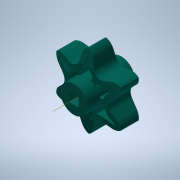
# Autodesk Inventor part: 276-2252.html
Saved by Autodesk Inventor 2020 (Build 240168000, 168)
## iProperties
Created: 2012-02-28
Part Number: 276-2252.html
Document SubType Name: Modeling
Designer: Autodesk Inc.
Density: 1.42 g/cm^3
Material: Acetal Resin, White
Catalog Web Link: http://www.vexrobotics.com/276-2252.html#
Vendor: VEX
Mass: 3.55844 g
Surface Area: 16.0324 cm^2
Volume: 2.50594 cm^3
Appearance: VEX Gears Green
Category: Motion
Company: Autodesk Inc.
Author: Autodesk Inc.
Autodesk Inventor part; units mm, degrees
ref_plane "YZ Plane" through (0, 0, 0) normal (1, 0, 0) x (0, 1, 0)
ref_plane "XZ Plane" through (0, 0, 0) normal (0, 1, 0) x (-1, 0, 0)
ref_plane "XY Plane" through (0, 0, 0) normal (0, 0, 1) x (1, 0, 0)
sketch "Sketch1" plane through (0, 0, 0) normal (0, 0, 1) x (1, 0, 0)
  arc A0 (-7.9913, 6.691) -> (-10.7412, 6.2014) centre (-8.8664, 3.639) ccw
  line L0 (-7.9913, 6.691) -> (-5.6103, 6.0082)
  arc A1 (-5.6103, 6.0082) -> (-2.3981, 7.8628) centre (-4.8997, 8.4865) ccw
  line L1 (-2.3981, 7.8628) -> (-1.7989, 10.2662)
  arc A2 (0, 12.4028) -> (-1.7989, 10.2662) centre (1.2818, 9.4981) ccw
  arc A3 (1.7989, 10.2662) -> (0, 12.4028) centre (-1.2818, 9.4981) ccw
  line L2 (1.7989, 10.2662) -> (2.3981, 7.8628)
  arc A4 (2.3981, 7.8628) -> (5.6103, 6.0082) centre (4.8997, 8.4865) ccw
  line L3 (5.6103, 6.0082) -> (7.9913, 6.691)
  arc A5 (10.7412, 6.2014) -> (7.9913, 6.691) centre (8.8664, 3.639) ccw
  arc A6 (9.7902, 3.5752) -> (10.7412, 6.2014) centre (7.5847, 5.8591) ccw
  line L4 (9.7902, 3.5752) -> (8.0084, 1.8545)
  arc A7 (8.0084, 1.8545) -> (8.0084, -1.8545) centre (9.7993, 0) ccw
  line L5 (8.0084, -1.8545) -> (9.7902, -3.5752)
  arc A8 (10.7412, -6.2014) -> (9.7902, -3.5752) centre (7.5847, -5.8591) ccw
  arc A9 (7.9913, -6.691) -> (10.7412, -6.2014) centre (8.8664, -3.639) ccw
  line L6 (7.9913, -6.691) -> (5.6103, -6.0082)
  arc A10 (5.6103, -6.0082) -> (2.3981, -7.8628) centre (4.8997, -8.4865) ccw
  line L7 (2.3981, -7.8628) -> (1.7989, -10.2662)
  arc A11 (0, -12.4028) -> (1.7989, -10.2662) centre (-1.2818, -9.4981) ccw
  arc A12 (-1.7989, -10.2662) -> (0, -12.4028) centre (1.2818, -9.4981) ccw
  line L8 (-1.7989, -10.2662) -> (-2.3981, -7.8628)
  arc A13 (-2.3981, -7.8628) -> (-5.6103, -6.0082) centre (-4.8997, -8.4865) ccw
  line L9 (-5.6103, -6.0082) -> (-7.9913, -6.691)
  arc A14 (-10.7412, -6.2014) -> (-7.9913, -6.691) centre (-8.8664, -3.639) ccw
  arc A15 (-9.7902, -3.5752) -> (-10.7412, -6.2014) centre (-7.5847, -5.8591) ccw
  line L10 (-9.7902, -3.5752) -> (-8.0084, -1.8545)
  arc A16 (-8.0084, -1.8545) -> (-8.0084, 1.8545) centre (-9.7993, 0) ccw
  line L11 (-8.0084, 1.8545) -> (-9.7902, 3.5752)
  arc A17 (-10.7412, 6.2014) -> (-9.7902, 3.5752) centre (-7.5847, 5.8591) ccw
  line L12 (-1.5875, 1.5875) -> (-1.5875, -1.5875)
  line L13 (-1.5875, -1.5875) -> (1.5875, -1.5875)
  line L14 (1.5875, -1.5875) -> (1.5875, 1.5875)
  line L15 (1.5875, 1.5875) -> (-1.5875, 1.5875)
  point P0 (0, 0)
  point P1 (0, 0)
  constraints: 36 point on circle, 32 end point, 18 centre point
extrude "Extrusion1" add sketch "Sketch1" along normal mid plane 7.62 contours L0 A1 L1 A2 A3 L2 A4 L3 A5 A6 L4 A7 L5 A8 A9 L6 A10 L7 A11 A12 L8 A13 L9 A14 A15 L10 A16 L11 A17 A0 | L15 L14 L13 L12
sketch "Sketch2" plane through (0, 0, 3.81) normal (0, 0, 1) x (1, 0, 0)
  circle A0 centre (0, 0) radius 4.4958
  dimension "d2" = 8.9916
  constraints: 1 centre point, 1 coincident
  measures "d2" diameter of A0
extrude "Extrusion2" add sketch "Sketch2" along normal blind 4.1402
mirror "Mirror1" about plane through (0, 0, 0) normal (0, 0, 1) of "Extrusion2"
extrude "Extrusion3" cut sketch "Sketch1" against normal up to surface (15.9004 mm away) from surface at 7.9502 contours L15 L14 L13 L12
sketch "Sketch3" plane through (0, 0, 3.81) normal (0, 0, 1) x (1, 0, 0)
  line L0 (-7.9913, 6.691) -> (-5.6103, 6.0082) projected
  arc A0 (-7.9913, 6.691) -> (-10.7412, 6.2014) centre (-8.8664, 3.639) ccw projected
  arc A1 (-10.7412, 6.2014) -> (-9.7902, 3.5752) centre (-7.5847, 5.8591) ccw projected
  line L1 (-8.0084, 1.8545) -> (-9.7902, 3.5752) projected
  arc A2 (-8.0084, -1.8545) -> (-8.0084, 1.8545) centre (-9.7993, 0) ccw projected
  line L2 (-9.7902, -3.5752) -> (-8.0084, -1.8545) projected
  arc A3 (-9.7902, -3.5752) -> (-10.7412, -6.2014) centre (-7.5847, -5.8591) ccw projected
  arc A4 (-10.7412, -6.2014) -> (-7.9913, -6.691) centre (-8.8664, -3.639) ccw projected
  line L3 (-5.6103, -6.0082) -> (-7.9913, -6.691) projected
  arc A5 (-2.3981, -7.8628) -> (-5.6103, -6.0082) centre (-4.8997, -8.4865) ccw projected
  line L4 (-1.7989, -10.2662) -> (-2.3981, -7.8628) projected
  arc A6 (-1.7989, -10.2662) -> (0, -12.4028) centre (1.2818, -9.4981) ccw projected
  arc A7 (0, -12.4028) -> (1.7989, -10.2662) centre (-1.2818, -9.4981) ccw projected
  line L5 (2.3981, -7.8628) -> (1.7989, -10.2662) projected
  arc A8 (5.6103, -6.0082) -> (2.3981, -7.8628) centre (4.8997, -8.4865) ccw projected
  line L6 (7.9913, -6.691) -> (5.6103, -6.0082) projected
  arc A9 (7.9913, -6.691) -> (10.7412, -6.2014) centre (8.8664, -3.639) ccw projected
  arc A10 (10.7412, -6.2014) -> (9.7902, -3.5752) centre (7.5847, -5.8591) ccw projected
  line L7 (8.0084, -1.8545) -> (9.7902, -3.5752) projected
  arc A11 (8.0084, 1.8545) -> (8.0084, -1.8545) centre (9.7993, 0) ccw projected
  line L8 (9.7902, 3.5752) -> (8.0084, 1.8545) projected
  arc A12 (9.7902, 3.5752) -> (10.7412, 6.2014) centre (7.5847, 5.8591) ccw projected
  arc A13 (10.7412, 6.2014) -> (7.9913, 6.691) centre (8.8664, 3.639) ccw projected
  line L9 (5.6103, 6.0082) -> (7.9913, 6.691) projected
  arc A14 (2.3981, 7.8628) -> (5.6103, 6.0082) centre (4.8997, 8.4865) ccw projected
  line L10 (1.7989, 10.2662) -> (2.3981, 7.8628) projected
  arc A15 (1.7989, 10.2662) -> (0, 12.4028) centre (-1.2818, 9.4981) ccw projected
  arc A16 (0, 12.4028) -> (-1.7989, 10.2662) centre (1.2818, 9.4981) ccw projected
  line L11 (-2.3981, 7.8628) -> (-1.7989, 10.2662) projected
  arc A17 (-5.6103, 6.0082) -> (-2.3981, 7.8628) centre (-4.8997, 8.4865) ccw projected
  circle A18 centre (0, 0) radius 5.0673 projected
  circle A19 centre (0, 0) radius 7.6454
  dimension "d8" = 15.2908
  constraints: 1 centre point, 1 coincident
  measures "d8" diameter of A19
sketch "Sketch4" plane through (0, 0, 0) normal (1, 0, 0) x (0, 1, 0)
  line L0 (7.6454, 3.81) -> (-7.6454, 3.81) projected
  line L1 (12.4028, 3.81) -> (12.4028, 2.9972)
  line L2 (12.4028, 2.9972) -> (7.6454, 3.81)
  line L3 (7.6454, 3.81) -> (12.4028, 3.81)
  line L4 (0, -0.762) -> (0, 4.572) projected
  point P0 (0, 0)
  dimension "d9" = 0.8128
  constraints: 6 end point
  measures "d9" distance of L1.start L1.end
revolve "Revolution1" cut sketch "Sketch4" angle 360 about axis through (0, 0, -10) along (0, 0, 1)
mirror "Mirror2" about plane through (0, 0, 0) normal (0, 0, 1) of "Revolution1"
sketch "Sketch5" plane through (0, 0, 3.81) normal (0, 0, 1) x (1, 0, 0)
  circle A0 centre (0, 0) radius 4.2
  line L0 (1.5875, 1.5875) -> (-1.5875, 1.5875)
  line L1 (1.5875, -1.5875) -> (1.5875, 1.5875)
  line L2 (-1.5875, -1.5875) -> (1.5875, -1.5875)
  line L3 (-1.5875, 1.5875) -> (-1.5875, -1.5875)
  line L4 (1.5875, -1.5875) -> (1.5875, 1.5875)
  line L5 (1.5875, 1.5875) -> (-1.5875, 1.5875)
  line L6 (-1.5875, 1.5875) -> (-1.5875, -1.5875)
  line L7 (-1.5875, -1.5875) -> (1.5875, -1.5875)
  circle A1 centre (0, 0) radius 4.2
  line L8 (9.0737, 4.9685) -> (7.2002, 3.1592)
  arc A2 (7.715, 1.5173) -> (7.2002, 3.1592) centre (0, 0) ccw
  spline S0 degree 3 poles (8.0084, 1.8545) (7.9726, 1.8199) (7.9378, 1.7843) (7.904, 1.7477) (7.8703, 1.7111) (7.8377, 1.6736) (7.8061, 1.6352) (7.7746, 1.5967) (7.7442, 1.5574) (7.715, 1.5173) knots 0 0 0 0 0.333333 0.333333 0.333333 0.666667 0.666667 0.666667 1 1 1 1
  line L9 (9.7902, 3.5752) -> (8.0084, 1.8545)
  spline S1 degree 3 poles (10.7537, 6.0542) (10.7649, 5.8724) (10.7604, 5.6896) (10.7402, 5.5082) (10.7201, 5.3269) (10.6842, 5.1472) (10.6331, 4.9717) (10.582, 4.7962) (10.5157, 4.6249) (10.435, 4.4605) (10.3544, 4.2961) (10.2594, 4.1386) (10.1514, 3.9902) (10.0434, 3.8419) (9.9224, 3.7029) (9.7902, 3.5752) knots 0 0 0 0 0.2 0.2 0.2 0.4 0.4 0.4 0.6 0.6 0.6 0.8 0.8 0.8 1 1 1 1
  ellipse E0 centre (10.4543, 6.0358) end of major axis (10.6042, 5.776) minor radius 0.2999 (10.7537, 6.0542) -> (10.6199, 6.2859) ccw
  spline S2 degree 3 poles (10.6199, 6.2859) (10.2987, 6.4986) (9.9401, 6.6495) (9.1019, 6.8432) (8.5734, 6.8415) (8.049, 6.7071) (8.0201, 6.6992) (7.9913, 6.691) knots 0 0 0 0 0.414162 0.414162 0.967573 0.967573 1 1 1 1
  spline S3 degree 3 poles (7.9913, 6.691) (7.7038, 6.6085) (7.144, 6.448) (6.3504, 6.2205) (5.8519, 6.0775) (5.6103, 6.0082) knots 0 0 0 0 0.333333 0.666667 1 1 1 1
  spline S4 degree 3 poles (5.1715, 5.9227) (5.2209, 5.928) (5.2701, 5.9346) (5.3192, 5.9427) (5.3682, 5.9508) (5.4171, 5.9603) (5.4656, 5.9712) (5.5141, 5.9822) (5.5624, 5.9945) (5.6103, 6.0082) knots 0 0 0 0 0.333333 0.333333 0.333333 0.666667 0.666667 0.666667 1 1 1 1
  arc A3 (6.3361, 4.6559) -> (5.1715, 5.9227) centre (0, 0) ccw
  spline S5 degree 3 poles (6.3361, 4.6559) (6.5468, 4.7163) (6.9811, 4.8409) (7.6702, 5.0385) (8.1556, 5.1776) (8.4048, 5.2491) knots 0 0 0 0 0.333333 0.666667 1 1 1 1
  spline S6 degree 3 poles (8.9441, 5.3122) (8.8534, 5.3164) (8.7624, 5.3132) (8.6721, 5.3027) (8.5819, 5.2921) (8.4923, 5.2742) (8.4048, 5.2491) knots 0 0 0 0 0.5 0.5 0.5 1 1 1 1
  spline S7 degree 3 poles (8.9441, 5.3122) (8.9583, 5.3115) (8.9723, 5.3093) (9.0099, 5.2995) (9.0348, 5.2877) (9.0777, 5.2549) (9.0957, 5.2339) (9.1211, 5.1896) (9.13, 5.1634) (9.1366, 5.1098) (9.1341, 5.0824) (9.1203, 5.0334) (9.1079, 5.0087) (9.0857, 4.9809) (9.0799, 4.9745) (9.0737, 4.9685) knots 0 0 0 0 0.091575 0.091575 0.26196 0.26196 0.432344 0.432344 0.602729 0.602729 0.773114 0.773114 0.945021 0.945021 1 1 1 1
  line L10 (5.549, -0.75) -> (4.6837, -0.75)
  arc A4 (5.8402, -0.9781) -> (5.549, -0.75) centre (5.549, -1.05) ccw
  arc A5 (5.8402, -0.9781) -> (6.9664, -2.9335) centre (9.7993, 0) ccw
  line L11 (7.2002, -3.1592) -> (6.9664, -2.9335)
  arc A6 (7.2002, -3.1592) -> (7.715, -1.5173) centre (0, 0) ccw
  arc A7 (7.715, 1.5173) -> (7.715, -1.5173) centre (9.7993, 0) ccw
  arc A8 (7.715, 1.5173) -> (7.2002, 3.1592) centre (0, 0) ccw
  line L12 (7.2002, 3.1592) -> (6.9664, 2.9335)
  arc A9 (6.9664, 2.9335) -> (5.8402, 0.9781) centre (9.7993, 0) ccw
  arc A10 (5.549, 0.75) -> (5.8402, 0.9781) centre (5.549, 1.05) ccw
  line L13 (4.6837, 0.75) -> (5.549, 0.75)
  arc A11 (4.391, 0.9844) -> (4.6837, 0.75) centre (4.6837, 1.05) ccw
  arc A12 (4.391, -0.9844) -> (4.391, 0.9844) centre (0, 0) ccw
  arc A13 (4.6837, -0.75) -> (4.391, -0.9844) centre (4.6837, -1.05) ccw
  spline S8 degree 3 poles (8.4048, -5.2491) (8.4923, -5.2742) (8.5818, -5.2921) (8.672, -5.3027) (8.7623, -5.3132) (8.8534, -5.3164) (8.9441, -5.3122) knots 0 0 0 0 0.5 0.5 0.5 1 1 1 1
  line L14 (8.4048, -5.2491) -> (6.3361, -4.6559)
  arc A14 (5.1715, -5.9227) -> (6.3361, -4.6559) centre (0, 0) ccw
  spline S9 degree 3 poles (5.6103, -6.0082) (5.5624, -5.9945) (5.5141, -5.9822) (5.4656, -5.9712) (5.4171, -5.9603) (5.3682, -5.9508) (5.3192, -5.9427) (5.2701, -5.9346) (5.2209, -5.928) (5.1715, -5.9227) knots 0 0 0 0 0.333333 0.333333 0.333333 0.666667 0.666667 0.666667 1 1 1 1
  line L15 (7.9913, -6.691) -> (5.6103, -6.0082)
  spline S10 degree 3 poles (10.6199, -6.2859) (10.2987, -6.4986) (9.9401, -6.6495) (9.1019, -6.8432) (8.5734, -6.8415) (8.049, -6.7071) (8.0201, -6.6992) (7.9913, -6.691) knots 0 0 0 0 0.414162 0.414162 0.967573 0.967573 1 1 1 1
  ellipse E1 centre (10.4543, -6.0358) end of major axis (10.3043, -6.2955) minor radius 0.2999 (10.6199, -6.2859) -> (10.7537, -6.0542) ccw
  spline S11 degree 3 poles (9.7902, -3.5752) (9.9224, -3.7029) (10.0434, -3.8419) (10.1514, -3.9903) (10.2594, -4.1386) (10.3544, -4.2961) (10.4351, -4.4605) (10.5157, -4.6249) (10.582, -4.7962) (10.6331, -4.9717) (10.6842, -5.1472) (10.7201, -5.3269) (10.7402, -5.5083) (10.7604, -5.6896) (10.7649, -5.8724) (10.7537, -6.0542) knots 0 0 0 0 0.2 0.2 0.2 0.4 0.4 0.4 0.6 0.6 0.6 0.8 0.8 0.8 1 1 1 1
  line L16 (9.7902, -3.5752) -> (8.0084, -1.8545)
  spline S12 degree 3 poles (7.715, -1.5173) (7.7442, -1.5574) (7.7746, -1.5967) (7.8061, -1.6352) (7.8377, -1.6736) (7.8703, -1.7111) (7.904, -1.7477) (7.9378, -1.7843) (7.9726, -1.8199) (8.0084, -1.8545) knots 0 0 0 0 0.333333 0.333333 0.333333 0.666667 0.666667 0.666667 1 1 1 1
  arc A15 (7.2002, -3.1592) -> (7.715, -1.5173) centre (0, 0) ccw
  spline S13 degree 3 poles (7.2002, -3.1592) (7.3872, -3.3398) (7.7753, -3.7147) (8.3989, -4.3169) (8.844, -4.7467) (9.0737, -4.9685) knots 0 0 0 0 0.333333 0.666667 1 1 1 1
  spline S14 degree 3 poles (9.0737, -4.9685) (9.0799, -4.9745) (9.0857, -4.9809) (9.1079, -5.0087) (9.1203, -5.0334) (9.1341, -5.0824) (9.1366, -5.1098) (9.13, -5.1634) (9.1211, -5.1896) (9.0957, -5.2339) (9.0777, -5.2549) (9.0348, -5.2877) (9.0099, -5.2995) (8.9723, -5.3093) (8.9583, -5.3115) (8.9441, -5.3122) knots 0 0 0 0 0.054979 0.054979 0.226886 0.226886 0.397271 0.397271 0.567656 0.567656 0.73804 0.73804 0.908425 0.908425 1 1 1 1
  arc A16 (1.343, -4.2949) -> (3.048, -3.3105) centre (0, 0) ccw
  arc A17 (1.6924, -4.4312) -> (1.343, -4.2949) centre (1.4325, -4.5812) ccw
  line L17 (2.125, -5.1806) -> (1.6924, -4.4312)
  arc A18 (2.0731, -5.5468) -> (2.125, -5.1806) centre (1.8652, -5.3306) ccw
  arc A19 (2.0731, -5.5468) -> (0.9427, -7.4999) centre (4.8997, -8.4865) ccw
  line L18 (0.8641, -7.8151) -> (0.9427, -7.4999)
  arc A20 (0.8641, -7.8151) -> (2.5435, -7.44) centre (0, 0) ccw
  arc A21 (5.1715, -5.9227) -> (2.5435, -7.44) centre (4.8997, -8.4865) ccw
  arc A22 (5.1715, -5.9227) -> (6.3361, -4.6559) centre (0, 0) ccw
  line L19 (6.3361, -4.6559) -> (6.0237, -4.5663)
  arc A23 (6.0237, -4.5663) -> (3.7671, -4.5688) centre (4.8997, -8.4865) ccw
  arc A24 (3.424, -4.4306) -> (3.7671, -4.5688) centre (3.6838, -4.2806) ccw
  line L20 (2.9914, -3.6812) -> (3.424, -4.4306)
  arc A25 (3.048, -3.3105) -> (2.9914, -3.6812) centre (3.2512, -3.5312) ccw
  spline S15 degree 3 poles (-0.3435, -9.9033) (-0.3233, -9.9842) (-0.2969, -10.064) (-0.2383, -10.2051) (-0.2078, -10.2671) (-0.1738, -10.3269) knots 0 0 0 0 0.548983 0.548983 1 1 1 1
  line L21 (-0.3435, -9.9033) -> (-0.8641, -7.8151)
  arc A26 (-2.5435, -7.44) -> (-0.8641, -7.8151) centre (0, 0) ccw
  spline S16 degree 3 poles (-2.3981, -7.8628) (-2.4102, -7.8144) (-2.4236, -7.7665) (-2.4384, -7.719) (-2.4533, -7.6715) (-2.4694, -7.6244) (-2.487, -7.5779) (-2.5045, -7.5314) (-2.5233, -7.4854) (-2.5435, -7.44) knots 0 0 0 0 0.333333 0.333333 0.333333 0.666667 0.666667 0.666667 1 1 1 1
  line L22 (-1.7989, -10.2662) -> (-2.3981, -7.8628)
  spline S17 degree 3 poles (-0.1338, -12.34) (-0.4786, -12.1683) (-0.7886, -11.9332) (-1.3754, -11.3041) (-1.6382, -10.8456) (-1.784, -10.3242) (-1.7917, -10.2952) (-1.7989, -10.2662) knots 0 0 0 0 0.414162 0.414162 0.967573 0.967573 1 1 1 1
  ellipse E2 centre (0, -12.0716) end of major axis (-0.2999, -12.0715) minor radius 0.2999 (-0.1338, -12.34) -> (0.1338, -12.34) ccw
  spline S18 degree 3 poles (0.1338, -12.34) (0.4786, -12.1683) (0.7886, -11.9332) (1.3754, -11.3041) (1.6382, -10.8456) (1.784, -10.3242) (1.7917, -10.2952) (1.7989, -10.2662) knots 0 0 0 0 0.414162 0.414162 0.967573 0.967573 1 1 1 1
  spline S19 degree 3 poles (1.7989, -10.2662) (1.8713, -9.9759) (2.0121, -9.4109) (2.2119, -8.6098) (2.3373, -8.1066) (2.3981, -7.8628) knots 0 0 0 0 0.333333 0.666667 1 1 1 1
  spline S20 degree 3 poles (2.5435, -7.44) (2.5233, -7.4854) (2.5045, -7.5314) (2.487, -7.5779) (2.4694, -7.6244) (2.4533, -7.6715) (2.4384, -7.719) (2.4236, -7.7665) (2.4102, -7.8144) (2.3981, -7.8628) knots 0 0 0 0 0.333333 0.333333 0.333333 0.666667 0.666667 0.666667 1 1 1 1
  arc A27 (0.8641, -7.8151) -> (2.5435, -7.44) centre (0, 0) ccw
  line L23 (0.8641, -7.8151) -> (0.3435, -9.9033)
  spline S21 degree 3 poles (0.1738, -10.3269) (0.2078, -10.2671) (0.2383, -10.2051) (0.2969, -10.064) (0.3233, -9.9842) (0.3435, -9.9033) knots 0 0 0 0 0.451017 0.451017 1 1 1 1
  spline S22 degree 3 poles (0.1738, -10.3269) (0.1621, -10.3473) (0.1468, -10.3657) (0.1289, -10.3808) (0.1109, -10.396) (0.0903, -10.4079) (0.0683, -10.4159) (0.0463, -10.4239) (0.023, -10.4279) (-0.0003, -10.4279) (-0.0236, -10.4279) (-0.0469, -10.4237) (-0.0688, -10.4157) (-0.0907, -10.4077) (-0.1112, -10.3958) (-0.129, -10.3807) (-0.1469, -10.3656) (-0.1622, -10.3473) (-0.1738, -10.3269) knots 0 0 0 0 0.166667 0.166667 0.166667 0.333333 0.333333 0.333333 0.5 0.5 0.5 0.666667 0.666667 0.666667 0.833333 0.833333 0.833333 1 1 1 1
  arc A28 (-3.048, -3.3105) -> (-1.343, -4.2949) centre (0, 0) ccw
  arc A29 (-2.9914, -3.6812) -> (-3.048, -3.3105) centre (-3.2512, -3.5312) ccw
  line L24 (-3.424, -4.4306) -> (-2.9914, -3.6812)
  arc A30 (-3.7671, -4.5688) -> (-3.424, -4.4306) centre (-3.6838, -4.2806) ccw
  arc A31 (-3.7671, -4.5688) -> (-6.0237, -4.5663) centre (-4.8997, -8.4865) ccw
  line L25 (-6.3361, -4.6559) -> (-6.0237, -4.5663)
  arc A32 (-6.3361, -4.6559) -> (-5.1715, -5.9227) centre (0, 0) ccw
  arc A33 (-2.5435, -7.44) -> (-5.1715, -5.9227) centre (-4.8997, -8.4865) ccw
  arc A34 (-2.5435, -7.44) -> (-0.8641, -7.8151) centre (0, 0) ccw
  line L26 (-0.8641, -7.8151) -> (-0.9427, -7.4999)
  arc A35 (-0.9427, -7.4999) -> (-2.0731, -5.5468) centre (-4.8997, -8.4865) ccw
  arc A36 (-2.125, -5.1806) -> (-2.0731, -5.5468) centre (-1.8652, -5.3306) ccw
  line L27 (-1.6924, -4.4312) -> (-2.125, -5.1806)
  arc A37 (-1.343, -4.2949) -> (-1.6924, -4.4312) centre (-1.4325, -4.5812) ccw
  line L28 (-9.0737, -4.9685) -> (-7.2002, -3.1592)
  arc A38 (-7.715, -1.5173) -> (-7.2002, -3.1592) centre (0, 0) ccw
  spline S23 degree 3 poles (-8.0084, -1.8545) (-7.9726, -1.8199) (-7.9378, -1.7843) (-7.904, -1.7477) (-7.8703, -1.7111) (-7.8377, -1.6736) (-7.8061, -1.6352) (-7.7746, -1.5967) (-7.7442, -1.5574) (-7.715, -1.5173) knots 0 0 0 0 0.333333 0.333333 0.333333 0.666667 0.666667 0.666667 1 1 1 1
  line L29 (-9.7902, -3.5752) -> (-8.0084, -1.8545)
  spline S24 degree 3 poles (-9.7902, -3.5752) (-9.9224, -3.7029) (-10.0434, -3.8419) (-10.1514, -3.9902) (-10.2594, -4.1386) (-10.3544, -4.2961) (-10.435, -4.4605) (-10.5157, -4.6249) (-10.582, -4.7962) (-10.6331, -4.9717) (-10.6842, -5.1471) (-10.7201, -5.3269) (-10.7402, -5.5082) (-10.7604, -5.6896) (-10.7649, -5.8724) (-10.7537, -6.0542) knots 0 0 0 0 0.2 0.2 0.2 0.4 0.4 0.4 0.6 0.6 0.6 0.8 0.8 0.8 1 1 1 1
  ellipse E3 centre (-10.4543, -6.0358) end of major axis (-10.3045, -6.2956) minor radius 0.2999 (-10.7537, -6.0542) -> (-10.6199, -6.2859) ccw
  spline S25 degree 3 poles (-10.6199, -6.2859) (-10.2987, -6.4986) (-9.9401, -6.6495) (-9.1019, -6.8432) (-8.5734, -6.8415) (-8.049, -6.7071) (-8.0201, -6.6992) (-7.9913, -6.691) knots 0 0 0 0 0.414162 0.414162 0.967573 0.967573 1 1 1 1
  spline S26 degree 3 poles (-7.9913, -6.691) (-7.7038, -6.6085) (-7.144, -6.448) (-6.3504, -6.2205) (-5.8519, -6.0775) (-5.6103, -6.0082) knots 0 0 0 0 0.333333 0.666667 1 1 1 1
  spline S27 degree 3 poles (-5.1715, -5.9227) (-5.2209, -5.928) (-5.2701, -5.9346) (-5.3192, -5.9427) (-5.3682, -5.9508) (-5.4171, -5.9603) (-5.4656, -5.9712) (-5.5141, -5.9822) (-5.5624, -5.9945) (-5.6103, -6.0082) knots 0 0 0 0 0.333333 0.333333 0.333333 0.666667 0.666667 0.666667 1 1 1 1
  arc A39 (-6.3361, -4.6559) -> (-5.1715, -5.9227) centre (0, 0) ccw
  spline S28 degree 3 poles (-6.3361, -4.6559) (-6.5468, -4.7163) (-6.9811, -4.8409) (-7.6702, -5.0385) (-8.1556, -5.1776) (-8.4048, -5.2491) knots 0 0 0 0 0.333333 0.666667 1 1 1 1
  spline S29 degree 3 poles (-8.9441, -5.3122) (-8.8534, -5.3164) (-8.7624, -5.3132) (-8.6721, -5.3027) (-8.5819, -5.2921) (-8.4923, -5.2742) (-8.4048, -5.2491) knots 0 0 0 0 0.5 0.5 0.5 1 1 1 1
  spline S30 degree 3 poles (-8.9441, -5.3122) (-8.9583, -5.3115) (-8.9723, -5.3093) (-9.0099, -5.2995) (-9.0348, -5.2877) (-9.0777, -5.2549) (-9.0957, -5.2339) (-9.1211, -5.1896) (-9.13, -5.1634) (-9.1366, -5.1098) (-9.1341, -5.0824) (-9.1203, -5.0334) (-9.1079, -5.0087) (-9.0857, -4.9809) (-9.0799, -4.9745) (-9.0737, -4.9685) knots 0 0 0 0 0.091575 0.091575 0.26196 0.26196 0.432344 0.432344 0.602729 0.602729 0.773114 0.773114 0.945021 0.945021 1 1 1 1
  arc A40 (-4.391, 0.9844) -> (-4.391, -0.9844) centre (0, 0) ccw
  arc A41 (-4.6837, 0.75) -> (-4.391, 0.9844) centre (-4.6837, 1.05) ccw
  line L30 (-5.549, 0.75) -> (-4.6837, 0.75)
  arc A42 (-5.8402, 0.9781) -> (-5.549, 0.75) centre (-5.549, 1.05) ccw
  arc A43 (-5.8402, 0.9781) -> (-6.9664, 2.9335) centre (-9.7993, 0) ccw
  line L31 (-7.2002, 3.1592) -> (-6.9664, 2.9335)
  arc A44 (-7.2002, 3.1592) -> (-7.715, 1.5173) centre (0, 0) ccw
  arc A45 (-7.715, -1.5173) -> (-7.715, 1.5173) centre (-9.7993, 0) ccw
  arc A46 (-7.715, -1.5173) -> (-7.2002, -3.1592) centre (0, 0) ccw
  line L32 (-7.2002, -3.1592) -> (-6.9664, -2.9335)
  arc A47 (-6.9664, -2.9335) -> (-5.8402, -0.9781) centre (-9.7993, 0) ccw
  arc A48 (-5.549, -0.75) -> (-5.8402, -0.9781) centre (-5.549, -1.05) ccw
  line L33 (-4.6837, -0.75) -> (-5.549, -0.75)
  arc A49 (-4.391, -0.9844) -> (-4.6837, -0.75) centre (-4.6837, -1.05) ccw
  spline S31 degree 3 poles (-8.4048, 5.2491) (-8.4849, 5.2721) (-8.5672, 5.2892) (-8.7187, 5.3089) (-8.7877, 5.3135) (-8.8564, 5.3139) knots 0 0 0 0 0.548983 0.548983 1 1 1 1
  line L34 (-8.4048, 5.2491) -> (-6.3361, 4.6559)
  arc A50 (-5.1715, 5.9227) -> (-6.3361, 4.6559) centre (0, 0) ccw
  spline S32 degree 3 poles (-5.6103, 6.0082) (-5.5624, 5.9945) (-5.5141, 5.9822) (-5.4656, 5.9712) (-5.4171, 5.9603) (-5.3682, 5.9508) (-5.3192, 5.9427) (-5.2701, 5.9346) (-5.2209, 5.928) (-5.1715, 5.9227) knots 0 0 0 0 0.333333 0.333333 0.333333 0.666667 0.666667 0.666667 1 1 1 1
  line L35 (-7.9913, 6.691) -> (-5.6103, 6.0082)
  spline S33 degree 3 poles (-10.6199, 6.2859) (-10.2987, 6.4986) (-9.9401, 6.6495) (-9.1019, 6.8432) (-8.5734, 6.8415) (-8.049, 6.7071) (-8.0201, 6.6992) (-7.9913, 6.691) knots 0 0 0 0 0.414162 0.414162 0.967573 0.967573 1 1 1 1
  ellipse E4 centre (-10.4543, 6.0358) end of major axis (-10.6044, 5.7761) minor radius 0.2999 (-10.6199, 6.2859) -> (-10.7537, 6.0542) ccw
  spline S34 degree 3 poles (-10.7537, 6.0542) (-10.7649, 5.8724) (-10.7604, 5.6896) (-10.7402, 5.5083) (-10.7201, 5.3269) (-10.6842, 5.1472) (-10.6331, 4.9717) (-10.582, 4.7962) (-10.5157, 4.625) (-10.4351, 4.4606) (-10.3544, 4.2962) (-10.2594, 4.1386) (-10.1514, 3.9903) (-10.0434, 3.8419) (-9.9224, 3.7029) (-9.7902, 3.5752) knots 0 0 0 0 0.2 0.2 0.2 0.4 0.4 0.4 0.6 0.6 0.6 0.8 0.8 0.8 1 1 1 1
  spline S35 degree 3 poles (-9.7902, 3.5752) (-9.575, 3.3674) (-9.1562, 2.9629) (-8.5623, 2.3894) (-8.1892, 2.0291) (-8.0084, 1.8545) knots 0 0 0 0 0.333333 0.666667 1 1 1 1
  spline S36 degree 3 poles (-7.715, 1.5173) (-7.7442, 1.5574) (-7.7746, 1.5967) (-7.8061, 1.6352) (-7.8377, 1.6736) (-7.8703, 1.7111) (-7.904, 1.7477) (-7.9378, 1.7843) (-7.9726, 1.8199) (-8.0084, 1.8545) knots 0 0 0 0 0.333333 0.333333 0.333333 0.666667 0.666667 0.666667 1 1 1 1
  arc A51 (-7.2002, 3.1592) -> (-7.715, 1.5173) centre (0, 0) ccw
  spline S37 degree 3 poles (-7.2002, 3.1592) (-7.3579, 3.3116) (-7.6828, 3.6254) (-8.1985, 4.1234) (-8.5618, 4.4741) (-8.7482, 4.6542) knots 0 0 0 0 0.333333 0.666667 1 1 1 1
  spline S38 degree 3 poles (-9.0302, 5.0129) (-8.9955, 4.9536) (-8.957, 4.8962) (-8.8642, 4.7749) (-8.8082, 4.7121) (-8.7482, 4.6542) knots 0 0 0 0 0.451017 0.451017 1 1 1 1
  spline S39 degree 3 poles (-9.0302, 5.0129) (-9.0421, 5.0333) (-9.0504, 5.0557) (-9.0545, 5.0788) (-9.0586, 5.1019) (-9.0586, 5.1257) (-9.0546, 5.1488) (-9.0505, 5.1718) (-9.0423, 5.1941) (-9.0307, 5.2142) (-9.019, 5.2344) (-9.0038, 5.2525) (-8.9859, 5.2674) (-8.968, 5.2823) (-8.9474, 5.2942) (-8.9254, 5.3021) (-8.9034, 5.31) (-8.88, 5.3141) (-8.8564, 5.3139) knots 0 0 0 0 0.166667 0.166667 0.166667 0.333333 0.333333 0.333333 0.5 0.5 0.5 0.666667 0.666667 0.666667 0.833333 0.833333 0.833333 1 1 1 1
  line L36 (-2.9914, 3.6812) -> (-3.424, 4.4306)
  arc A52 (-3.048, 3.3105) -> (-2.9914, 3.6812) centre (-3.2512, 3.5312) ccw
  arc A53 (-1.6911, 4.4272) -> (-1.3418, 4.2909) centre (-1.4313, 4.5772) ccw
  line L37 (-2.1237, 5.1766) -> (-1.6911, 4.4272)
  arc A54 (-2.0718, 5.5428) -> (-2.1237, 5.1766) centre (-1.8639, 5.3266) ccw
  arc A55 (-2.0718, 5.5428) -> (-0.9414, 7.4959) centre (-4.8984, 8.4825) ccw
  arc A56 (-5.1715, 5.9227) -> (-2.5435, 7.44) centre (-4.8997, 8.4865) ccw
  arc A57 (-5.1715, 5.9227) -> (-6.3361, 4.6559) centre (0, 0) ccw
  line L38 (-6.3361, 4.6559) -> (-6.0237, 4.5663)
  arc A58 (-6.0237, 4.5663) -> (-3.7671, 4.5688) centre (-4.8997, 8.4865) ccw
  arc A59 (-3.424, 4.4306) -> (-3.7671, 4.5688) centre (-3.6838, 4.2806) ccw
  spline S40 degree 3 poles (0.3422, 9.8993) (0.3224, 9.9809) (0.2963, 10.0614) (0.238, 10.2038) (0.2077, 10.2665) (0.1738, 10.3269) knots 0 0 0 0 0.548983 0.548983 1 1 1 1
  line L39 (0.3422, 9.8993) -> (0.9414, 7.4959)
  spline S41 degree 3 poles (2.3981, 7.8628) (2.4102, 7.8144) (2.4236, 7.7665) (2.4384, 7.719) (2.4533, 7.6715) (2.4694, 7.6244) (2.487, 7.5779) (2.5045, 7.5314) (2.5233, 7.4854) (2.5435, 7.44) knots 0 0 0 0 0.333333 0.333333 0.333333 0.666667 0.666667 0.666667 1 1 1 1
  line L40 (1.7989, 10.2662) -> (2.3981, 7.8628)
  spline S42 degree 3 poles (0.1338, 12.34) (0.4786, 12.1683) (0.7886, 11.9332) (1.3754, 11.3041) (1.6382, 10.8456) (1.784, 10.3242) (1.7917, 10.2952) (1.7989, 10.2662) knots 0 0 0 0 0.414162 0.414162 0.967573 0.967573 1 1 1 1
  ellipse E5 centre (0, 12.0716) end of major axis (-0.2999, 12.0717) minor radius 0.2999 (0.1338, 12.34) -> (-0.1338, 12.34) ccw
  spline S43 degree 3 poles (-0.1338, 12.34) (-0.4786, 12.1683) (-0.7886, 11.9332) (-1.3754, 11.3041) (-1.6382, 10.8456) (-1.784, 10.3242) (-1.7917, 10.2952) (-1.7989, 10.2662) knots 0 0 0 0 0.414162 0.414162 0.967573 0.967573 1 1 1 1
  spline S44 degree 3 poles (-1.7989, 10.2662) (-1.8713, 9.9759) (-2.0121, 9.4109) (-2.2119, 8.6098) (-2.3373, 8.1066) (-2.3981, 7.8628) knots 0 0 0 0 0.333333 0.666667 1 1 1 1
  spline S45 degree 3 poles (-2.5435, 7.44) (-2.5233, 7.4854) (-2.5045, 7.5314) (-2.487, 7.5779) (-2.4694, 7.6244) (-2.4533, 7.6715) (-2.4384, 7.719) (-2.4236, 7.7665) (-2.4102, 7.8144) (-2.3981, 7.8628) knots 0 0 0 0 0.333333 0.333333 0.333333 0.666667 0.666667 0.666667 1 1 1 1
  line L41 (-0.9414, 7.4959) -> (-0.3422, 9.8993)
  spline S46 degree 3 poles (-0.1738, 10.3269) (-0.2077, 10.2665) (-0.238, 10.2038) (-0.2963, 10.0614) (-0.3224, 9.9809) (-0.3422, 9.8993) knots 0 0 0 0 0.451017 0.451017 1 1 1 1
  spline S47 degree 3 poles (-0.1738, 10.3269) (-0.1621, 10.3473) (-0.1468, 10.3657) (-0.1289, 10.3808) (-0.1109, 10.396) (-0.0903, 10.4079) (-0.0683, 10.4159) (-0.0463, 10.4239) (-0.023, 10.4279) (0.0003, 10.4279) (0.0236, 10.4279) (0.0469, 10.4237) (0.0688, 10.4157) (0.0907, 10.4077) (0.1112, 10.3958) (0.129, 10.3807) (0.1469, 10.3656) (0.1622, 10.3473) (0.1738, 10.3269) knots 0 0 0 0 0.166667 0.166667 0.166667 0.333333 0.333333 0.333333 0.5 0.5 0.5 0.666667 0.666667 0.666667 0.833333 0.833333 0.833333 1 1 1 1
  line L42 (1.6911, 4.4272) -> (2.1237, 5.1766)
  arc A60 (1.3418, 4.2909) -> (1.6911, 4.4272) centre (1.4313, 4.5772) ccw
  arc A61 (2.9914, 3.6812) -> (3.048, 3.3105) centre (3.2512, 3.5312) ccw
  line L43 (3.424, 4.4306) -> (2.9914, 3.6812)
  arc A62 (3.7671, 4.5688) -> (3.424, 4.4306) centre (3.6838, 4.2806) ccw
  arc A63 (3.7671, 4.5688) -> (6.0237, 4.5663) centre (4.8997, 8.4865) ccw
  line L44 (6.3361, 4.6559) -> (6.0237, 4.5663)
  arc A64 (6.3361, 4.6559) -> (5.1715, 5.9227) centre (0, 0) ccw
  arc A65 (2.5435, 7.44) -> (5.1715, 5.9227) centre (4.8997, 8.4865) ccw
  arc A66 (0.9414, 7.4959) -> (2.0718, 5.5428) centre (4.8984, 8.4825) ccw
  arc A67 (2.1237, 5.1766) -> (2.0718, 5.5428) centre (1.8639, 5.3266) ccw
  arc A68 (7.543, 1.2472) -> (4.8516, 5.9088) centre (0, 0) ccw
  arc A69 (1.3418, 4.2909) -> (-1.3418, 4.2909) centre (0, 0) ccw
  constraints: 134 point on circle, 90 end point, 69 centre point, 1 coincident, 1 tangent, 138 other
extrude "Extrusion4" cut sketch "Sketch5" against normal blind 2.8194 contours L37 A54 A55 L41 S46 S47 S40 L39 A66 A67 L42 A60 A69 A53
pattern_circular "Circular Pattern1" count 6 over 360 about axis through (0, 0, 3.81) along (0, 0, 1) of "Extrusion4"
mirror "Mirror3" about plane through (0, 0, 0) normal (0, 0, 1) of "Extrusion4", "Circular Pattern1"
sketch "Sketch6" plane through (0, 0, 7.9502) normal (0, 0, 1) x (1, 0, 0)
  circle A0 centre (0, 0) radius 4.4958 projected
  circle A1 centre (0, 0) radius 1.5875
  constraints: 1 centre point, 1 coincident
surface extrude "ExtrusionSrf1" sketch "Sketch6" against normal up to surface (15.9004 mm away) shown no curves A1
body "Solid1"
body "Srf1"
